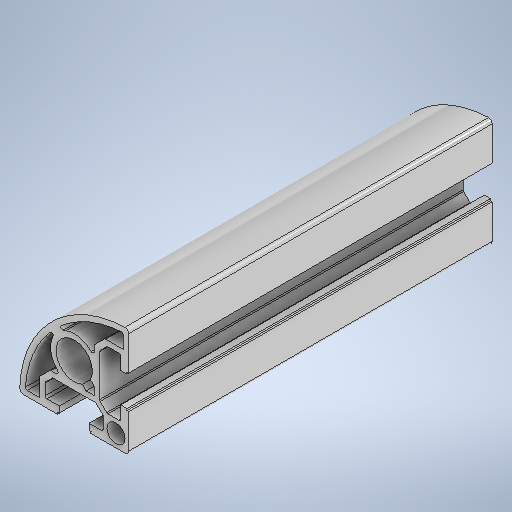
# Autodesk Inventor part: Perfil 30×30 R90 2 rasgos_001
Saved by Autodesk Inventor 2026 (Build 300175000, 175)
## iProperties
Created: 2025-04-06
Part Number: Perfil 30×30 R90 2 rasgos_001
Material: Aluminum 6061
Document SubType Name: Modeling
Designer: Tony Dias
Density: 2.7 g/cm^3
Appearance: Aluminum - Polished
Author: Tony Dias
Autodesk Inventor part; units mm, degrees
ref_plane "YZ Plane" through (0, 0, 0) normal (1, 0, 0) x (0, 1, 0)
ref_plane "XZ Plane" through (0, 0, 0) normal (0, 1, 0) x (-1, 0, 0)
ref_plane "XY Plane" through (0, 0, 0) normal (0, 0, 1) x (1, 0, 0)
sketch "Sketch1" plane through (0, 0, 0) normal (0, 0, 1) x (1, 0, 0)
  line L0 (-30, 0) -> (0, 0) construction
  circle A0 centre (-15, 15) radius 5 construction
  line L1 (-30, 30) -> (0, 0) construction
  line L2 (0, 0) -> (-10.9, 0) construction
  line L3 (-10.9, 2.2) -> (-10.9, 0) construction
  circle A1 centre (-3.5, 3.5) radius 2.5 construction
  line L4 (-12.7399, 10.5399) -> (-11.7, 9.5)
  line L5 (-11.7, 9.5) -> (-9.5, 9.5)
  arc A2 (-18.5355, 18.5355) -> (-12.7399, 10.5399) centre (-15, 15) ccw
  line L6 (-10.9, 2.2) -> (-7, 2.2)
  arc A3 (-5.2678, 5.2678) -> (-1.7322, 1.7322) centre (-3.5, 3.5) ccw
  line L7 (-1.7322, 1.7322) -> (0, 0)
  line L8 (-5.2678, 5.2678) -> (-9.5, 9.5)
  line L9 (-9.0607, 8) -> (-7, 5.9393)
  line L10 (-7, 5.9393) -> (-7, 2.2)
  line L11 (-9.0607, 8) -> (-15, 8)
  line L12 (-30, 0) -> (-19.1, 0) construction
  line L13 (-15, 15) -> (-15, 0) construction
  line L14 (-19.1, 2.2) -> (-19.1, 0) construction
  line L15 (-19.1, 2.2) -> (-23, 2.2)
  line L16 (-23, 5.9393) -> (-23, 2.2)
  line L17 (-20.9393, 8) -> (-23, 5.9393)
  line L18 (-20.9393, 8) -> (-15, 8)
  line L19 (-28.4605, 1.5) -> (-24.5, 1.5)
  circle A4 centre (0, 0) radius 30 construction
  circle A5 centre (0, 0) radius 28.5 construction
  line L20 (-24.5, 1.5) -> (-24.5, 6.5607)
  line L21 (-21.5607, 9.5) -> (-24.5, 6.5607)
  line L22 (-21.5607, 9.5) -> (-18.4641, 9.5)
  arc A6 (-21.2132, 21.2132) -> (-30, 0) centre (0, 0) ccw
  line L23 (-21.2132, 21.2132) -> (-18.5355, 18.5355)
  arc A7 (-21.0782, 17.3034) -> (-18.4641, 9.5) centre (-15, 15) ccw
  arc A8 (-21.648, 18.5368) -> (-28.4605, 1.5) centre (0, 0) ccw
  arc A9 (-20.8009, 18.0339) -> (-21.648, 18.5368) centre (-21.2683, 18.2116) ccw
  arc A10 (-20.8009, 18.0339) -> (-21.0782, 17.3034) centre (633.4955, -230.7557) ccw
  line L24 (-19.1, 0) -> (-19.6, 0) construction
  line L25 (-19.6, 0) -> (-19.6, 0.5)
  line L26 (-19.6, 0.5) -> (-19.1, 0.5)
  line L27 (-19.1, 0.5) -> (-19.1, 0) construction
  line L28 (-19.1, 0.5) -> (-19.1, 2.2)
  line L29 (-30, 0) -> (-19.6, 0)
  line L30 (-10.9, 0) -> (-10.4, 0) construction
  line L31 (-10.4, 0) -> (-10.4, 0.5)
  line L32 (-10.4, 0.5) -> (-10.9, 0.5)
  line L33 (-10.9, 0.5) -> (-10.9, 0) construction
  line L34 (-10.9, 2.2) -> (-10.9, 0.5)
  line L35 (-10.4, 0) -> (0, 0)
  dimension "d0" = 30
  dimension "d1" = 10
  dimension "d2" = 15
  dimension "d3" = 15
  dimension "d4" = 4.1
  dimension "d5" = 2.2
  dimension "d6" = 5
  dimension "d8" = 2.2
  dimension "d10" = 0.75
  dimension "d12" = 11.5
  dimension "d13" = 1
  dimension "d14" = 8
  dimension "d15" = 4.1
  dimension "d16" = 1.5
  dimension "d17" = 1.5
  dimension "d18" = 1.5
  dimension "d19" = 1.5
  dimension "d25" = 1.5
  dimension "d35" = 1.5
  dimension "d36" = 2.2
  dimension "d37" = 0.5
  dimension "d39" = 700
  dimension "d41" = 0.5
  constraints: 70 end point, 22 point on circle, 11 centre point, 10 horizontal, 7 equal length, 6 concentric, 6 parallel, 5 vertical, 4 collinear, 3 coincident, 3 tangent, 2 horizontal alignment, 2 perpendicular, 2 point on line, 1 midpoint, 1 vertical alignment, 13 other
  measures "d0" distance of L0.start L0.end
  measures "d1" diameter of A0
  measures "d2" horizontal distance of point (0, 0) A0.centre
  measures "d3" horizontal distance of point (0, 0) A0.centre
  measures "d4" horizontal distance of A0.centre L2.end
  measures "d5" distance of L3.start L2.end
  measures "d6" diameter of A1
  measures "d8" distance of L4.end L5.end
  measures "d10" distance of the line from the sketch origin of L9
  measures "d12" horizontal distance of A0.centre A3.centre
  measures "d13" distance edge to line of A3 L10
  measures "d14" vertical distance of L2.end L9.start
  measures "d15" horizontal distance of L13.start L12.end
  measures "d16" distance between parallel lines of L0 L19
  measures "d17" radial gap between concentric circles of A5 A4
  measures "d18" distance between parallel lines of L16 L20
  measures "d19" distance between parallel lines of L17 L21
  measures "d25" distance between parallel lines of L18 L22
  measures "d35" radial gap between concentric circles of A0 A7
  measures "d37" radius of A9
  measures "d39" radius of A10
  measures "d41" distance of L24.end L25.end
extrude "Extrusion1" add sketch "Sketch1" along normal mid plane 100
fillet "Fillet2" radius 1 1 edges at (-30, 0, 0)
fillet "Fillet3" radius 0.5 10 edges at (-28.4605, 1.5, 0) (-23, 2.2, 0) (-24.5, 6.5607, 0) (-21.5607, 9.5, 0) (-18.4641, 9.5, 0) (-23, 5.9393, 0) (-20.9393, 8, 0) (-9.0607, 8, 0) (-7, 5.9393, 0) (-7, 2.2, 0)
mirror "Mirror2" about plane through (-5.2678, 5.2678, 0) normal (0.7071068, 0.7071068, 0) of "Extrusion1", "Fillet2", "Fillet3"
fillet "Fillet4" radius 1 1 edges at (0, 0, 0)
equation "\"d3\" = d2"
equation "\"d8\" = d5"
equation "\"d15\" = d4"
equation "\"d17\" = d16"
body "Solid1"
